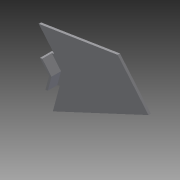
# Autodesk Inventor part: Right Bicep
Saved by Autodesk Inventor 2014 SP2 (Build 180246200, 246)
## iProperties
Created: 2015-08-01
Part Number: Right Bicep
Material: Generic
Document SubType Name: Modeling
Designer: Devon
Density: 1 g/cm^3
Appearance: Default
Author: Devon
Autodesk Inventor part; units mm, degrees
ref_plane "YZ Plane" through (0, 0, 0) normal (1, 0, 0) x (0, 1, 0)
ref_plane "XZ Plane" through (0, 0, 0) normal (0, 1, 0) x (-1, 0, 0)
ref_plane "XY Plane" through (0, 0, 0) normal (0, 0, 1) x (1, 0, 0)
sketch "Sketch1" plane through (0, 0, 0) normal (0, 0, 1) x (1, 0, 0)
  line L0 (-10.4788, 3.5567) -> (22.1748, -35.3584)
  line L1 (-10.4788, 3.5567) -> (40.3212, 3.5567) construction
  line L2 (22.1748, -35.3584) -> (8.205, -87.4942)
  line L3 (8.205, -87.4942) -> (134.8162, -28.4545)
  line L4 (134.8162, -28.4545) -> (93.9992, 20.1894)
  line L5 (93.9992, 20.1894) -> (-10.4788, 3.5567)
  point P0 (0, 0)
  dimension "d0" = 50.8
  dimension "d1" = 50
  dimension "d2" = 53.975
  dimension "d3" = 125
  dimension "d4" = 139.7
  dimension "d5" = 50
  dimension "d6" = 63.5
  dimension "d7" = 75
  constraints: 12 end point, 1 equal length, 1 horizontal, 1 parallel
  measures "d0" distance of L0.start L0.end
  measures "d1" angle of L0 L1
  measures "d2" distance of L0.end L2.end
  measures "d3" angle of L0 L2
  measures "d4" distance of L2.end L3.end
  measures "d5" angle of L3 L2
  measures "d6" distance of L3.end L4.end
  measures "d7" angle of L4 L3
extrude "Extrusion1" add sketch "Sketch1" along normal blind 3.175
sketch "Sketch2" plane through (0, 0, 3.175) normal (0, 0, 1) x (1, 0, 0)
  line L0 (-10.4788, 3.5567) -> (22.1748, -35.3584) projected
  line L1 (22.1748, -35.3584) -> (8.205, -87.4942) projected
  line L2 (22.1748, -35.3584) -> (9.9297, -20.7652)
  line L3 (22.1748, -35.3584) -> (17.2443, -53.7593)
  line L4 (9.9297, -20.7652) -> (3.7302, -22.1396)
  line L5 (17.2443, -53.7593) -> (11.0448, -55.1337)
  line L6 (15.9753, -36.7328) -> (3.7302, -22.1396)
  line L7 (15.9753, -36.7328) -> (11.0448, -55.1337)
  point P0 (0, 0)
  dimension "d10" = 19.05
  dimension "d11" = 19.05
  dimension "d12" = 6.35
  dimension "d13" = 6.35
  dimension "d14" = 6.35
  constraints: 12 end point, 2 point on line, 1 parallel
  measures "d10" distance of L0.end L2.end
  measures "d11" distance of L0.end L3.end
  measures "d12" distance of L2.end L4.end
  measures "d13" distance of L3.end L5.end
  measures "d14" distance of L0.end L6.start
extrude "Extrusion2" add sketch "Sketch2" against normal blind 3.175
sketch "Sketch3" plane through (0, 0, 3.175) normal (0, 0, 1) x (1, 0, 0)
  line L0 (9.9297, -20.7652) -> (3.7302, -22.1396) projected
  line L1 (3.7302, -22.1396) -> (15.9753, -36.7328) projected
  line L2 (15.9753, -36.7328) -> (11.0448, -55.1337) projected
  line L3 (11.0448, -55.1337) -> (17.2443, -53.7593) projected
  line L4 (11.0448, -55.1337) -> (14.1446, -54.4465)
  line L5 (3.7302, -22.1396) -> (6.83, -21.4524)
  line L6 (19.0751, -36.0456) -> (6.83, -21.4524)
  line L7 (19.0751, -36.0456) -> (14.1446, -54.4465)
  point P0 (0, 0)
  dimension "d17" = 3.175
  dimension "d18" = 3.175
  dimension "d19" = 3.175
  constraints: 8 end point, 2 midpoint
  measures "d17" distance of L2.end L4.end
  measures "d18" distance of L0.end L5.end
  measures "d19" distance of L1.end L6.start
extrude "Extrusion3" add sketch "Sketch3" along normal blind 12.7
body "Solid1"
